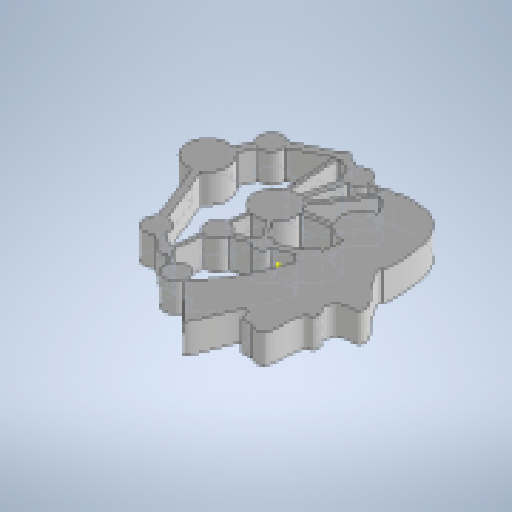
# Autodesk Inventor part: logotipo
Saved by Autodesk Inventor 2024.1 (Build 281209000, 209)
## iProperties
Created: 2021-05-16
Part Number: logotipo
Material: Genérico
Document SubType Name: Modeling
Designer: ander
Density: 1 g/cm^3
Appearance: Valor por defecto
Author: ander
## iProperties of the stored document _3DPrint.ipt
Created: 2023-02-08
Part Number: _3DPrint
Material: Generic
Document SubType Name: Modeling
Designer: jonathan.zea
Density: 1 g/cm^3
Appearance: Default
Author: jonathan.zea
Autodesk Inventor part; units mm, degrees
ref_plane "YZ Plane" through (0, 0, 0) normal (1, 0, 0) x (0, 1, 0)
ref_plane "XZ Plane" through (0, 0, 0) normal (0, 1, 0) x (-1, 0, 0)
ref_plane "XY Plane" through (0, 0, 0) normal (0, 0, 1) x (1, 0, 0)
sketch "Boceto1" plane through (0, 0, 0) normal (0, 1, 0) x (-1, 0, 0)
  line L0 (0.7571, 0.1512) -> (0.1707, 0.7175)
  line L1 (-0.3154, 0.2141) -> (-0.5066, 0.2141)
  line L2 (-0.5066, 0.2141) -> (-0.7019, 0.3122) construction
  line L3 (-0.7019, 0.3122) -> (-0.7706, 0.1635) construction
  line L4 (-0.7706, 0.1635) -> (-0.7706, -0.0789) construction
  line L5 (-0.7706, -0.0789) -> (-0.7706, -0.1081) construction
  line L6 (-0.7706, -0.1081) -> (-0.7706, -0.0789) construction
  line L7 (-0.7706, -0.0789) -> (-0.7706, -0.4444) construction
  line L8 (-0.7706, -0.4444) -> (-0.9222, -0.394) construction
  line L9 (-0.9222, -0.394) -> (-0.9222, -0.4977) construction
  line L10 (-0.9222, -0.4977) -> (-0.8857, -0.4977) construction
  line L11 (-0.8857, -0.4977) -> (-0.9222, -0.4977) construction
  line L12 (-0.9222, -0.4977) -> (-0.9222, -0.5852) construction
  line L13 (-0.9222, -0.5852) -> (-0.8465, -0.5852) construction
  line L14 (-0.8465, -0.5852) -> (-0.8465, -0.8863) construction
  line L15 (-0.8465, -0.8863) -> (-1.188, -0.8863) construction
  line L16 (-1.188, -0.8863) -> (-1.2326, -0.8863) construction
  line L17 (-1.2326, -0.8863) -> (-1.279, -1.0804) construction
  line L18 (-1.279, -1.0804) -> (-1.0359, -1.2388) construction
  line L19 (-1.0359, -1.2388) -> (-0.7506, -1.6783) construction
  line L20 (-0.7506, -1.6783) -> (-0.7706, -1.7281) construction
  line L21 (-0.7706, -1.7281) -> (-0.8168, -1.7372) construction
  spline S0 degree 4 poles (-0.5066, 0.2141) (-0.7019, 0.3122) (-0.7706, 0.1635) (-0.7706, -0.0789) (-0.7706, -0.1081) (-0.7706, -0.0789) (-0.7706, -0.4444) (-0.9222, -0.394) (-0.9222, -0.4977) (-0.9222, -0.4977) (-0.8857, -0.4977) (-0.9222, -0.4977) (-0.9222, -0.5852) (-0.9222, -0.5852) (-0.8465, -0.5852) (-0.8465, -0.8863) (-1.188, -0.8863) (-1.2326, -0.8863) (-1.279, -1.0804) (-1.0359, -1.2388) (-0.7506, -1.6783) (-0.7706, -1.7281) (-0.8168, -1.7372) (-0.8168, -1.7372) knots 1 1 1 1 1 2 3 4 5 6 7 8 9 10 11 12 13 14 15 16 17 18 19 20 21 21 21 21 21
  spline S1 degree 3 poles (0.1707, 0.7175) (0.0754, 0.9968) (-0.2135, -0.4775) (-0.3154, 0.2141) knots 0 0 0 0 1 1 1 1
  line L22 (0.2371, -2.7708) -> (0.3067, -2.7764) construction
  arc A0 (1.6232, -0.3484) -> (1.6486, -0.3122) centre (1.7988, -0.4443) ccw
  line L23 (0.7432, 0.1021) -> (0.4849, -0.1382) construction
  line L24 (1.4257, -0.2424) -> (1.6232, -0.3484)
  line L25 (1.4533, -0.2043) -> (1.6486, -0.3122)
  line L26 (1.2616, -0.1542) -> (1.0892, -0.0616)
  line L27 (1.1191, -0.0183) -> (1.28, -0.1073)
  line L28 (1.2968, -0.2429) -> (1.2417, -0.7117)
  line L29 (1.2993, -0.7293) -> (1.3595, -0.2662)
  line L30 (1.2504, -1.106) -> (1.2062, -1.446)
  line L31 (1.195, -1.1088) -> (1.157, -1.4319)
  line L32 (0.3817, -2.9301) -> (0.5867, -2.9301)
  line L33 (0.4005, -2.8782) -> (0.5894, -2.8782)
  line L34 (1.1346, -3.0902) -> (0.96, -3.0116)
  line L35 (0.9788, -2.9646) -> (1.1448, -3.0394)
  line L36 (1.2335, -2.0915) -> (1.2845, -3.0066)
  line L37 (1.1766, -2.1135) -> (1.2254, -2.9887)
  line L38 (1.0262, -2.1206) -> (0.8841, -2.7315)
  line L39 (0.928, -2.0872) -> (0.7839, -2.7066)
  line L40 (0.7645, -1.9146) -> (0.3067, -1.999)
  line L41 (0.2575, -1.9312) -> (0.7418, -1.8418)
  circle A1 centre (2.4049, -1.9339) radius 0.35
  circle A2 centre (2.0549, -2.6758) radius 0.2
  spline S2 degree 4 poles (0.066, -2.5131) (0.1124, -2.6328) (0.1707, -2.721) (0.2371, -2.7708) (0.3067, -2.7764) knots 0 0 0 0 0 1 1 1 1 1
  line L42 (-0.0327, -1.743) -> (-0.034, -1.8209) construction
  line L43 (0.1707, -2.721) -> (0.2371, -2.7708) construction
  line L44 (0.1124, -2.6328) -> (0.1707, -2.721) construction
  line L45 (0.066, -2.5131) -> (0.1124, -2.6328) construction
  arc A3 (0.2607, -2.9652) -> (0.3817, -2.9301) centre (0.3005, -2.8762) ccw
  arc A4 (0.4005, -2.8782) -> (0.3713, -2.8056) centre (0.3005, -2.8762) ccw
  arc A5 (0.5867, -2.9301) -> (0.96, -3.0116) centre (0.7874, -2.9066) ccw
  arc A6 (0.9788, -2.9646) -> (0.8841, -2.7315) centre (0.7874, -2.9066) ccw
  arc A7 (0.7839, -2.7066) -> (0.5894, -2.8782) centre (0.7874, -2.9066) ccw
  arc A8 (1.1346, -3.0902) -> (1.2845, -3.0066) centre (1.2319, -3.0885) ccw
  arc A9 (1.2254, -2.9887) -> (1.1448, -3.0394) centre (1.2319, -3.0885) ccw
  arc A10 (1.0262, -2.1206) -> (1.1766, -2.1135) centre (1.0852, -1.7744) ccw
  arc A11 (0.066, -2.5131) -> (0.3067, -1.999) centre (0.0009, -2.1692) ccw
  arc A12 (0.2575, -1.9312) -> (-0.034, -1.8209) centre (0.0009, -2.1692) ccw
  arc A13 (1.2335, -2.0915) -> (1.2062, -1.446) centre (1.0852, -1.7744) ccw
  arc A14 (1.2616, -0.1542) -> (1.2968, -0.2429) centre (1.3609, -0.1661) ccw
  arc A15 (1.3595, -0.2662) -> (1.4257, -0.2424) centre (1.3609, -0.1661) ccw
  arc A16 (1.4533, -0.2043) -> (1.28, -0.1073) centre (1.3609, -0.1661) ccw
  arc A17 (1.2504, -1.106) -> (1.2993, -0.7293) centre (1.213, -0.9096) ccw
  arc A18 (1.1191, -0.0183) -> (0.7571, 0.1512) centre (0.9411, 0.0727) ccw
  arc A19 (0.7432, 0.1021) -> (1.0892, -0.0616) centre (0.9411, 0.0727) ccw
  line L46 (-0.8168, -1.7372) -> (-0.8465, -2.225) construction
  line L47 (-0.8465, -2.225) -> (-0.7342, -2.7579) construction
  line L48 (-0.7342, -2.7579) -> (-0.5513, -3.0392) construction
  line L49 (-0.5513, -3.0392) -> (0.066, -3.0392) construction
  line L50 (0.066, -3.0392) -> (0.2607, -2.9652) construction
  spline S3 degree 4 poles (-0.8168, -1.7372) (-0.8465, -2.225) (-0.7342, -2.7579) (-0.5513, -3.0392) (0.066, -3.0392) (0.2607, -2.9652) knots 1 1 1 1 1 2 3 3 3 3 3
  line L51 (1.0259, -0.9802) -> (0.7633, -1.0896)
  line L52 (1.0144, -0.8863) -> (0.7354, -1.0025)
  line L53 (0.5076, -1.196) -> (0.1835, -1.331)
  line L54 (0.4633, -1.0896) -> (0.168, -1.2125)
  arc A20 (1.2417, -0.7117) -> (1.0144, -0.8863) centre (1.213, -0.9096) ccw
  arc A21 (1.0259, -0.9802) -> (1.195, -1.1088) centre (1.213, -0.9096) ccw
  arc A22 (0.7354, -1.0025) -> (0.4633, -1.0896) centre (0.6133, -1.0896) ccw
  spline S4 degree 4 poles (0.7432, 0.1021) (0.4849, -0.1382) (0.2873, -0.4446) (0.149, -0.7798) (0.0634, -1.1119) knots 0 0 0 0 0 1 1 1 1 1
  spline S5 degree 4 poles (-0.0104, -1.4964) (-0.0211, -1.5802) (-0.0285, -1.6626) (-0.0327, -1.743) (-0.034, -1.8209) knots 0 0 0 0 0 1 1 1 1 1
  line L55 (0.4849, -0.1382) -> (0.2873, -0.4446) construction
  line L56 (0.2873, -0.4446) -> (0.149, -0.7798) construction
  line L57 (0.149, -0.7798) -> (0.0634, -1.1119) construction
  line L58 (-0.0285, -1.6626) -> (-0.0327, -1.743) construction
  line L59 (-0.0211, -1.5802) -> (-0.0285, -1.6626) construction
  line L60 (-0.0104, -1.4964) -> (-0.0211, -1.5802) construction
  arc A23 (0.168, -1.2125) -> (0.0634, -1.1119) centre (-0.0135, -1.2965) ccw
  arc A24 (-0.0104, -1.4964) -> (0.1835, -1.331) centre (-0.0135, -1.2965) ccw
  line L61 (0.7299, -1.1838) -> (0.92, -1.4659)
  line L62 (0.8612, -1.5055) -> (0.6735, -1.2269)
  arc A25 (1.157, -1.4319) -> (0.92, -1.4659) centre (1.0852, -1.7744) ccw
  arc A26 (0.8612, -1.5055) -> (0.7418, -1.8418) centre (1.0852, -1.7744) ccw
  arc A27 (0.5076, -1.196) -> (0.6735, -1.2269) centre (0.6133, -1.0896) ccw
  arc A28 (0.7299, -1.1838) -> (0.7633, -1.0896) centre (0.6133, -1.0896) ccw
  line L63 (0.8843, -2.061) -> (0.3713, -2.8056)
  line L64 (0.8311, -2.0152) -> (0.3067, -2.7764)
  arc A29 (0.7645, -1.9146) -> (0.8311, -2.0152) centre (1.0852, -1.7744) ccw
  arc A30 (0.8843, -2.061) -> (0.928, -2.0872) centre (1.0852, -1.7744) ccw
  point P0 (0.112, 0.7334)
  point P1 (-0.1906, 0.061)
  point P2 (-0.9222, -1.4293)
  point P3 (-0.9222, -1.4293)
  constraints: 58 point on circle, 56 end point, 31 centre point, 9 parallel, 7 point on line, 6 coincident, 6 horizontal, 6 vertical, 22 other
sketch "Boceto2" plane through (0, 0, 0) normal (0, 1, 0) x (-1, 0, 0)
  point P0 (0, 0)
sketch "Boceto3" plane through (0, 0, 0) normal (0, 1, 0) x (-1, 0, 0)
  point P0 (0, 0)
extrude "Extrusión1" add sketch "Boceto1" along normal blind 0.5
sketch "Sketch4" plane through (0, 0, 0) normal (0, -1, 0) x (1, 0, 0)
  circle A0 centre (-2.4049, -1.9339) radius 0.35 projected
  circle A1 centre (-2.0549, -2.6758) radius 0.2 projected
  line L0 (-0.7571, 0.1512) -> (-0.1707, 0.7175) projected
  arc A2 (-0.7571, 0.1512) -> (-1.1191, -0.0183) centre (-0.9411, 0.0727) ccw projected
  line L1 (-1.28, -0.1073) -> (-1.1191, -0.0183) projected
  arc A3 (-1.28, -0.1073) -> (-1.4533, -0.2043) centre (-1.3609, -0.1661) ccw projected
  line L2 (-1.6486, -0.3122) -> (-1.4533, -0.2043) projected
  arc A4 (-1.6486, -0.3122) -> (-1.6232, -0.3484) centre (-1.7988, -0.4443) ccw projected
  line L3 (-1.4257, -0.2424) -> (-1.6232, -0.3484) projected
  arc A5 (-1.4257, -0.2424) -> (-1.3595, -0.2662) centre (-1.3609, -0.1661) ccw projected
  line L4 (-1.2993, -0.7293) -> (-1.3595, -0.2662) projected
  arc A6 (-1.2993, -0.7293) -> (-1.2504, -1.106) centre (-1.213, -0.9096) ccw projected
  line L5 (-1.2062, -1.446) -> (-1.2504, -1.106) projected
  arc A7 (-1.2062, -1.446) -> (-1.2335, -2.0915) centre (-1.0852, -1.7744) ccw projected
  line L6 (-1.2845, -3.0066) -> (-1.2335, -2.0915) projected
  arc A8 (-1.2845, -3.0066) -> (-1.1346, -3.0902) centre (-1.2319, -3.0885) ccw projected
  line L7 (-0.96, -3.0116) -> (-1.1346, -3.0902) projected
  arc A9 (-0.96, -3.0116) -> (-0.5867, -2.9301) centre (-0.7874, -2.9066) ccw projected
  line L8 (-0.3817, -2.9301) -> (-0.5867, -2.9301) projected
  arc A10 (-0.3817, -2.9301) -> (-0.2607, -2.9652) centre (-0.3005, -2.8762) ccw projected
  line L9 (0.3154, 0.2141) -> (0.5066, 0.2141) projected
  arc A11 (-0.1835, -1.331) -> (0.0104, -1.4964) centre (0.0135, -1.2965) ccw projected
  ellipse E0 centre (-0.7198, -1.4697) end of major axis (-0.4566, -2.9445) minor radius 0.718 (0.034, -1.8209) -> (0.0104, -1.4964) ccw projected
  arc A12 (0.034, -1.8209) -> (-0.2575, -1.9312) centre (-0.0009, -2.1692) ccw projected
  line L10 (-0.7418, -1.8418) -> (-0.2575, -1.9312) projected
  arc A13 (-0.7418, -1.8418) -> (-0.8612, -1.5055) centre (-1.0852, -1.7744) ccw projected
  line L11 (-0.6735, -1.2269) -> (-0.8612, -1.5055) projected
  arc A14 (-0.6735, -1.2269) -> (-0.5076, -1.196) centre (-0.6133, -1.0896) ccw projected
  line L12 (-0.1835, -1.331) -> (-0.5076, -1.196) projected
  line L13 (-0.8311, -2.0152) -> (-0.3067, -2.7764) projected
  arc A15 (-0.8311, -2.0152) -> (-0.7645, -1.9146) centre (-1.0852, -1.7744) ccw projected
  line L14 (-0.3067, -1.999) -> (-0.7645, -1.9146) projected
  arc A16 (-0.3067, -1.999) -> (-0.066, -2.5131) centre (-0.0009, -2.1692) ccw projected
  ellipse E1 centre (-0.3332, -1.8674) end of major axis (-0.3155, -2.7768) minor radius 0.3644 (-0.3067, -2.7764) -> (-0.066, -2.5131) ccw projected
  arc A17 (-1.1766, -2.1135) -> (-1.0262, -2.1206) centre (-1.0852, -1.7744) ccw projected
  line L15 (-0.8841, -2.7315) -> (-1.0262, -2.1206) projected
  arc A18 (-0.8841, -2.7315) -> (-0.9788, -2.9646) centre (-0.7874, -2.9066) ccw projected
  line L16 (-1.1448, -3.0394) -> (-0.9788, -2.9646) projected
  arc A19 (-1.1448, -3.0394) -> (-1.2254, -2.9887) centre (-1.2319, -3.0885) ccw projected
  line L17 (-1.1766, -2.1135) -> (-1.2254, -2.9887) projected
  arc A20 (-0.928, -2.0872) -> (-0.8843, -2.061) centre (-1.0852, -1.7744) ccw projected
  line L18 (-0.3713, -2.8056) -> (-0.8843, -2.061) projected
  arc A21 (-0.3713, -2.8056) -> (-0.4005, -2.8782) centre (-0.3005, -2.8762) ccw projected
  line L19 (-0.5894, -2.8782) -> (-0.4005, -2.8782) projected
  arc A22 (-0.5894, -2.8782) -> (-0.7839, -2.7066) centre (-0.7874, -2.9066) ccw projected
  line L20 (-0.928, -2.0872) -> (-0.7839, -2.7066) projected
  arc A23 (-1.195, -1.1088) -> (-1.0259, -0.9802) centre (-1.213, -0.9096) ccw projected
  line L21 (-0.7633, -1.0896) -> (-1.0259, -0.9802) projected
  arc A24 (-0.7633, -1.0896) -> (-0.7299, -1.1838) centre (-0.6133, -1.0896) ccw projected
  line L22 (-0.92, -1.4659) -> (-0.7299, -1.1838) projected
  arc A25 (-0.92, -1.4659) -> (-1.157, -1.4319) centre (-1.0852, -1.7744) ccw projected
  line L23 (-1.195, -1.1088) -> (-1.157, -1.4319) projected
  line L24 (-1.2968, -0.2429) -> (-1.2417, -0.7117) projected
  arc A26 (-1.2968, -0.2429) -> (-1.2616, -0.1542) centre (-1.3609, -0.1661) ccw projected
  line L25 (-1.0892, -0.0616) -> (-1.2616, -0.1542) projected
  arc A27 (-1.0892, -0.0616) -> (-0.7432, 0.1021) centre (-0.9411, 0.0727) ccw projected
  arc A28 (-0.0634, -1.1119) -> (-0.168, -1.2125) centre (0.0135, -1.2965) ccw projected
  line L26 (-0.4633, -1.0896) -> (-0.168, -1.2125) projected
  arc A29 (-0.4633, -1.0896) -> (-0.7354, -1.0025) centre (-0.6133, -1.0896) ccw projected
  line L27 (-1.0144, -0.8863) -> (-0.7354, -1.0025) projected
  arc A30 (-1.0144, -0.8863) -> (-1.2417, -0.7117) centre (-1.213, -0.9096) ccw projected
  line L28 (-0.7874, -2.9066) -> (-1.2319, -3.0885)
  line L29 (-1.2319, -3.0885) -> (-2.0549, -2.6758)
  line L30 (-2.0549, -2.6758) -> (-2.4049, -1.9339)
  line L31 (-2.4049, -1.9339) -> (-1.7988, -0.4443)
  arc A31 (-1.28, -0.1073) -> (-1.4533, -0.2043) centre (-1.3609, -0.1661) ccw projected
  line L32 (-1.7988, -0.4443) -> (-1.3609, -0.1661)
  line L33 (-1.3944, -0.1134) -> (-1.8492, -0.4022)
  line L34 (-1.8492, -0.4022) -> (-2.4731, -1.9357)
  line L35 (-2.4731, -1.9357) -> (-2.1022, -2.722)
  line L36 (-2.1022, -2.722) -> (-1.2345, -3.1571)
  line L37 (-1.2345, -3.1571) -> (-0.7637, -2.9645)
  line L38 (-1.3274, -0.2189) -> (-1.7484, -0.4863)
  line L39 (-1.7484, -0.4863) -> (-2.3367, -1.932)
  line L40 (-2.3367, -1.932) -> (-2.0076, -2.6296)
  line L41 (-2.0076, -2.6296) -> (-1.2293, -3.0199)
  line L42 (-1.2293, -3.0199) -> (-0.811, -2.8488)
  line L43 (-0.7637, -2.9645) -> (-0.811, -2.8488)
  line L44 (-1.3274, -0.2189) -> (-1.3944, -0.1134)
  point P0 (0, 0)
  dimension "d23" = 0.125
  dimension "d26" = 0.125
  constraints: 34 end point, 2 midpoint, 2 perpendicular, 1 parallel, 14 other
  measures "d23" distance between parallel lines of L36 L41
  measures "d26" distance between parallel lines of L37 L42
extrude "Extrusion2" [suppressed]
scale "Scale1" factors (5, 5, 5) then translate (1.3822, -2, 5.0541) bodies 1
equation "\"height\" = 0.5"
